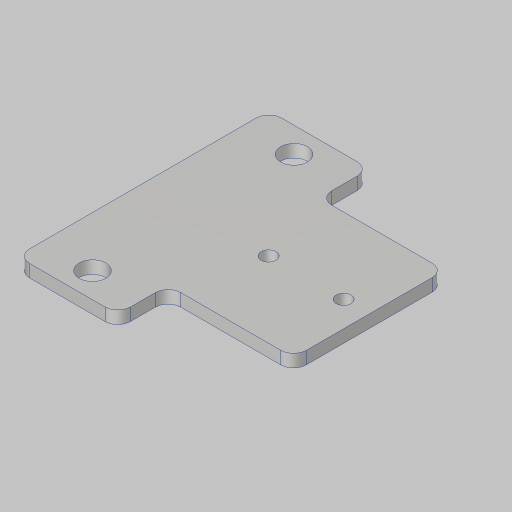
# Autodesk Inventor part: DB1-010
Saved by Autodesk Inventor 2023.5 (Build 275446000, 446)
## iProperties
Created: 2025-01-31
Part Number: DB1-010
Material: Aluminum 6061
Document SubType Name: Modeling
Designer: slick
Density: 2.7 g/cm^3
Appearance: Aluminum - Flat
Author: slick
Autodesk Inventor part; units mm, degrees
ref_plane "YZ Plane" through (0, 0, 0) normal (1, 0, 0) x (0, 1, 0)
ref_plane "XZ Plane" through (0, 0, 0) normal (0, 1, 0) x (-1, 0, 0)
ref_plane "XY Plane" through (0, 0, 0) normal (0, 0, 1) x (1, 0, 0)
sketch "Sketch1" plane through (0, 0, 0) normal (0, 1, 0) x (-1, 0, 0)
  line L0 (-12.7, -31.75) -> (12.7, -31.75)
  line L1 (12.7, -31.75) -> (12.7, 31.75)
  line L2 (12.7, 31.75) -> (-12.7, 31.75)
  line L3 (-12.7, 31.75) -> (-12.7, -31.75)
  line L4 (-12.7, -31.75) -> (12.7, 31.75) construction
  line L5 (12.7, -31.75) -> (-12.7, 31.75) construction
  line L6 (-12.7, 19.05) -> (-44.323, 19.05)
  line L7 (-44.323, 19.05) -> (-44.323, -19.05)
  line L8 (-44.323, -19.05) -> (-12.7, -19.05)
  point P0 (0, 0)
  dimension "d0" = 25.4
  dimension "d1" = 63.5
  dimension "d21" = 31.623
  dimension "d22" = 12.7
  dimension "d23" = 12.7
  constraints: 18 end point, 3 perpendicular, 2 horizontal, 2 midpoint, 2 parallel, 2 point on line
  measures "d0" distance of L1.end L2.end
  measures "d1" distance of L0.end L1.end
  measures "d21" distance of L6.start L6.end
  measures "d22" distance between parallel lines of L2 L6
  measures "d23" distance between parallel lines of L0 L8
extrude "Extrusion1" add sketch "Sketch1" along normal blind 3.175
sketch "Sketch2" plane through (0, 3.175, 0) normal (0, 1, 0) x (1, 0, 0)
  line L0 (0, -25.4) -> (0, 25.4) construction
  line L1 (-12.7, 31.75) -> (-12.7, -31.75) construction
  point P0 (0, 0)
  point P1 (0, 0)
  dimension "d4" = 50.8
  constraints: 2 end point, 2 vertical alignment, 1 coincident, 1 midpoint, 1 vertical
  measures "d4" distance of L0.start L0.end
hole "Hole1" at (0, 3.175, 25.4) at (0, 3.175, -25.4) direction (0, -1, 0) diameter 6.7564 end through all clearance for "Flat Head Machine Screw (82)" size "1/4" standard "Ansi Unified Screw Threads"
sketch "Sketch3" plane through (0, 3.175, 0) normal (0, 1, 0) x (1, 0, 0)
  line L0 (44.323, -19.05) -> (44.323, 19.05) construction
  point P0 (0, 0)
  point P1 (18.9813, 0)
  point P2 (37.8968, 0)
  point P3 (0, 0)
  dimension "d13" = 18.9155
  dimension "d24" = 6.4262
  constraints: 2 horizontal alignment, 1 coincident
  measures "d13" distance of point (18.981, 0) point (37.897, 0)
  measures "d24" distance from line of L0 point (37.897, 0)
hole "Hole2" at (18.9813, 3.175, 0) at (37.8968, 3.175, 0) direction (0, -1, 0) diameter 3.81 end through all clearance for "Flat Head Machine Screw (82)" size "#6" standard "Ansi Unified Screw Threads"
fillet "Fillet1" radius 3.175 8 edges at (12.7, 1.5875, 19.05) (12.7, 1.5875, 31.75) (-12.7, 1.5875, 31.75) (-12.7, 1.5875, -31.75) (12.7, 1.5875, -31.75) (12.7, 1.5875, -19.05) (44.323, 1.5875, -19.05) (44.323, 1.5875, 19.05)
body "Solid1"
